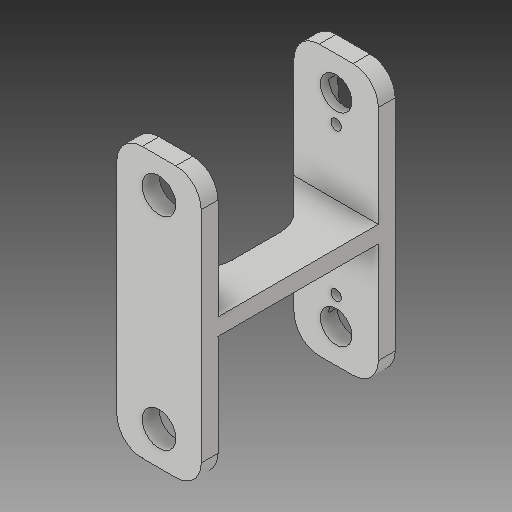
# Autodesk Inventor part: v5_femur
Saved by Autodesk Inventor 2019 (Build 230136000, 136)
## iProperties
Created: 2019-02-03
Part Number: v5_femur
Material: Generic
Document SubType Name: Modeling
Designer: Daniel
Density: 1 g/cm^3
Appearance: Default
Author: Daniel
Autodesk Inventor part; units mm, degrees
note: some values were not read from the file. Chosen so that the rebuilt part matches the saved one: direction of "Hole1"; direction of "Hole4"; direction of "Hole5"; direction of "Hole6"; direction of "Hole7".
ref_plane "YZ Plane" through (0, 0, 0) normal (1, 0, 0) x (0, 1, 0)
ref_plane "XZ Plane" through (0, 0, 0) normal (0, 1, 0) x (-1, 0, 0)
ref_plane "XY Plane" through (0, 0, 0) normal (0, 0, 1) x (1, 0, 0)
sketch "Sketch1" plane through (0, 0, 0) normal (0, 1, 0) x (-1, 0, 0)
  line L0 (14, 0) -> (-14, 0) projected
  line L1 (0, -32.2) -> (0, 32.2) projected
  line L2 (10, 23) -> (-10, 23)
  line L3 (-10, 23) -> (-10, -23)
  line L4 (-10, -23) -> (10, -23)
  line L5 (10, -23) -> (10, 23)
  point P0 (0, 0)
  dimension "d0" = 46
  dimension "d1" = 20
  constraints: 8 end point, 2 parallel, 1 horizontal, 1 perpendicular, 2 other
  measures "d0" distance between parallel lines of L4 L2
  measures "d1" distance between parallel lines of L3 L5
extrude "Extrusion1" add sketch "Sketch1" along normal blind 4
sketch "Sketch2" plane through (0, 4, 0) normal (0, 1, 0) x (1, 0, 0)
  line L0 (-10, -23) -> (10, -23) projected
  line L1 (10, -23) -> (10, 23) projected
  line L2 (10, 23) -> (-10, 23) projected
  line L3 (-10, 23) -> (-10, -23) projected
  line L4 (-10, -23) -> (10, -23)
  line L5 (10, -23) -> (10, -19)
  line L6 (10, -19) -> (-10, -19)
  line L7 (-10, -19) -> (-10, -23)
  line L8 (-10, 19) -> (10, 19)
  line L9 (10, 19) -> (10, 23)
  line L10 (10, 23) -> (-10, 23)
  line L11 (-10, 23) -> (-10, 19)
  line L12 (-10, -23) -> (10, -23) projected
  line L13 (-10, 23) -> (-10, -23) projected
  line L14 (10, -23) -> (10, 23) projected
  line L15 (10, 23) -> (-10, 23) projected
  point P0 (0, 0)
  dimension "d4" = 4
  dimension "d5" = 4
  constraints: 16 end point, 4 collinear, 4 parallel, 2 horizontal, 2 perpendicular, 2 point on line
  measures "d4" distance between parallel lines of L0 L6
  measures "d5" distance between parallel lines of L2 L8
extrude "Extrusion2" add sketch "Sketch2" along normal blind 30 contours L3 L6 L1 L0 | L3 L2 L1 L8
sketch "Sketch4" plane through (-10, 0, 23) normal (0, 0, 1) x (1, 0, 0)
  line L0 (0, 0) -> (20, 0) projected
  line L1 (20, 0) -> (20, 34) projected
  line L2 (0, 34) -> (20, 34) projected
  line L3 (0, 0) -> (0, 34) projected
  point P0 (10, 0)
  point P1 (10, 26)
  dimension "d8" = 10
  dimension "d9" = 8
  measures "d8" distance from line of L3 point (10, 26)
  measures "d9" distance from line of L2 point (10, 26)
hole "Hole1" at (0, 26, 23) direction (0, 0, -1) diameter 8 depth 42
sketch "Sketch10" plane through (10, 0, -23) normal (0, 0, -1) x (-1, 0, 0)
  line L0 (0, 34) -> (20, 34) projected
  line L1 (0, 0) -> (0, 34) projected
  line L2 (0, 0) -> (20, 0) projected
  line L3 (20, 0) -> (20, 34) projected
  circle A0 centre (10, 26) radius 4 projected
  circle A1 centre (10, 26) radius 3.75
  circle A2 centre (10, 12) radius 2.5
  line L4 (-6.7241, 9.5) -> (37.2046, 9.5) construction
  line L5 (6.25, 26) -> (7.5505, 11.5)
  line L6 (13.75, 26) -> (12.4495, 11.5)
  point P0 (10, 0)
  dimension "d47" = 16.5
  dimension "d48" = 7.5
  dimension "d49" = 5
  dimension "d50" = 10
  dimension "d51" = 2
  dimension "d52" = 2
  dimension "d53" = 8
  dimension "d54" = 8
  constraints: 6 end point, 4 point on circle, 2 centre point, 1 coincident, 1 horizontal, 1 tangent
  measures "d47" distance from line of L4 A1.centre
  measures "d48" diameter of A1
  measures "d49" diameter of A2
  measures "d50" distance from line of L1 A2.centre
  measures "d51" distance from line of L4 L6.end
  measures "d52" distance from line of L4 L5.end
  measures "d53" distance from line of L0 L6.start
  measures "d54" distance from line of L0 L5.start
extrude "Extrusion4" cut sketch "Sketch10" against normal blind 2 contours L5 A1 L6 A0 | A0 L6 A2 L5 | L5 A1 L6 | A2 L6 L5 picked at (10.4522, 22.2104)
sketch "Sketch11" plane through (10, 0, -21) normal (0, 0, -1) x (-1, 0, 0)
  line L0 (7.5505, 11.5) -> (6.25, 26) projected
  arc A0 (7.5505, 11.5) -> (12.4495, 11.5) centre (10, 12) ccw projected
  line L1 (13.75, 26) -> (12.4495, 11.5) projected
  arc A1 (13.75, 26) -> (6.25, 26) centre (10, 26) ccw projected
  point P0 (10, 0)
  constraints: 1 coincident
hole "Hole4" at (0, 26, -21) direction (0, 0, 1) diameter 7.5 depth 40
sketch "Sketch12" plane through (10, 0, -21) normal (0, 0, -1) x (-1, 0, 0)
  arc A0 (6.3099, 25.3327) -> (13.6901, 25.3327) centre (10, 26) ccw projected
  line L0 (7.5505, 11.5) -> (6.3099, 25.3327) projected
  arc A1 (7.5505, 11.5) -> (12.4495, 11.5) centre (10, 12) ccw projected
  line L1 (13.6901, 25.3327) -> (12.4495, 11.5) projected
  line L2 (0, 0) -> (0, 34) projected
  point P0 (10, 0)
  point P1 (10, 19.5)
  point P2 (0, 28)
  dimension "d64" = 6.5
  dimension "d65" = 10
  measures "d64" distance of A0.centre point (10, 19.5)
  measures "d65" distance from line of L2 point (10, 19.5)
hole "Hole5" at (0, 19.5, -21) direction (0, 0, 1) diameter 2.5 depth 40
sketch "Sketch13" plane through (0, 0, 0) normal (0, -1, 0) x (1, 0, 0)
  line L0 (-10, 23) -> (10, 23) projected
  line L1 (-10, -23) -> (-10, 23) projected
  line L2 (10, -23) -> (-10, -23) projected
  line L3 (10, 23) -> (10, -23) projected
  line L4 (10, 23) -> (10, -23) projected
  line L5 (-10, -19) -> (-10, 19) projected
  line L6 (10, 23) -> (-10, 23)
  line L7 (-10, 23) -> (-10, 19)
  line L8 (-10, 19) -> (10, 19)
  line L9 (10, 19) -> (10, 23)
  line L10 (10, -23) -> (-10, -23)
  line L11 (-10, -23) -> (-10, -19)
  line L12 (-10, -19) -> (10, -19)
  line L13 (10, -19) -> (10, -23)
  point P0 (0, 0)
  constraints: 16 end point, 4 parallel, 2 horizontal, 2 perpendicular
extrude "Extrusion5" add sketch "Sketch13" along normal blind 30 contours L0 L3 L8 L1 | L12 L3 L2 L1
sketch "Sketch14" plane through (10, 34, -23) normal (0, 0, -1) x (-1, 0, 0)
  arc A0 (7.5505, -22.5) -> (12.4495, -22.5) centre (10, -22) ccw projected
  line L0 (7.5505, -22.5) -> (6.25, -8) projected
  arc A1 (13.75, -8) -> (6.25, -8) centre (10, -8) ccw projected
  line L1 (13.75, -8) -> (12.4495, -22.5) projected
  line L2 (20, -64) -> (20, 0) projected
  line L3 (0, 0) -> (20, 0) projected
  line L4 (0, -64) -> (0, 0) projected
  line L5 (20, -64) -> (0, -64) projected
  line L6 (0, -34) -> (0, -64) projected
  line L7 (0, -40) -> (20, -40) construction
  circle A2 centre (10, -56) radius 3.75
  circle A3 centre (10, -42.5) radius 2.5
  line L8 (6.25, -56) -> (7.5505, -42)
  line L9 (13.75, -56) -> (12.4495, -42)
  point P0 (10, -34)
  dimension "d77" = 8
  dimension "d78" = 10
  dimension "d79" = 7.5
  dimension "d80" = 16
  dimension "d81" = 5
  dimension "d82" = 10
  dimension "d85" = 2
  dimension "d86" = 8
  dimension "d87" = 2
  dimension "d88" = 8
  constraints: 6 end point, 4 point on circle, 2 centre point, 2 point on line, 1 horizontal, 1 tangent
  measures "d77" distance from line of L5 A2.centre
  measures "d78" distance from line of L2 A2.centre
  measures "d79" diameter of A2
  measures "d80" distance from line of L7 A2.centre
  measures "d81" diameter of A3
  measures "d82" distance from line of L2 A3.centre
  measures "d85" distance from line of L7 L8.end
  measures "d86" distance from line of L5 L8.start
  measures "d87" distance from line of L7 L9.end
  measures "d88" distance from line of L5 L9.start
extrude "Extrusion6" cut sketch "Sketch14" against normal blind 2 contours L8 A2 L9 | L8 A3 L9 A2 | L8 A3 L9
sketch "Sketch15" plane through (10, 34, -21) normal (0, 0, -1) x (-1, 0, 0)
  arc A0 (6.25, -56) -> (13.75, -56) centre (10, -56) ccw projected
  line L0 (12.4495, -42) -> (13.75, -56) projected
  arc A1 (12.4495, -42) -> (7.5505, -42) centre (10, -42.5) ccw projected
  line L1 (6.25, -56) -> (7.5505, -42) projected
  point P0 (10, -34)
  constraints: 1 coincident
hole "Hole6" at (0, -22, -21) direction (0, 0, 1) diameter 7.5 depth 40
sketch "Sketch16" plane through (10, 34, -21) normal (0, 0, -1) x (-1, 0, 0)
  arc A0 (13.6858, -55.3093) -> (6.3142, -55.3093) centre (10, -56) ccw projected
  line L0 (12.4495, -42) -> (13.6858, -55.3093) projected
  arc A1 (12.4495, -42) -> (7.5505, -42) centre (10, -42.5) ccw projected
  line L1 (6.3142, -55.3093) -> (7.5505, -42) projected
  line L2 (12.4495, -42) -> (13.75, -56) projected
  arc A2 (6.25, -56) -> (13.75, -56) centre (10, -56) ccw projected
  line L3 (6.25, -56) -> (7.5505, -42) projected
  arc A3 (12.4495, -42) -> (7.5505, -42) centre (10, -42.5) ccw projected
  arc A4 (7.5505, -22.5) -> (12.4495, -22.5) centre (10, -22) ccw projected
  line L4 (7.5505, -22.5) -> (6.25, -8) projected
  arc A5 (13.75, -8) -> (6.25, -8) centre (10, -8) ccw projected
  line L5 (13.75, -8) -> (12.4495, -22.5) projected
  line L6 (20, -64) -> (20, 0) projected
  line L7 (0, 0) -> (20, 0) projected
  line L8 (0, -64) -> (0, 0) projected
  line L9 (20, -64) -> (0, -64) projected
  point P0 (10, -34)
  point P1 (10, -49.5)
  dimension "d98" = 10
  dimension "d99" = 6.5
  measures "d98" distance from line of L8 point (10, -49.5)
  measures "d99" distance of A0.centre point (10, -49.5)
hole "Hole7" at (0, -15.5, -21) direction (0, 0, 1) diameter 2.5 end up to surface
sketch "Sketch17" plane through (-10, 34, 23) normal (0, 0, 1) x (1, 0, 0)
  line L0 (20, -64) -> (0, -64) projected
  line L1 (20, -64) -> (20, 0) projected
  point P0 (10, -34)
  point P1 (10, -56)
  dimension "d107" = 8
  dimension "d108" = 10
  measures "d107" distance from line of L0 point (10, -56)
  measures "d108" distance from line of L1 point (10, -56)
hole "Hole8" at (0, -22, 23) direction (0, 0, -1) diameter 8 depth 4
fillet "Fillet4" radius 6 8 edges at (10, -30, -21) (-10, -30, -21) (10, -30, 21) (-10, -30, 21) (10, 34, 21) (10, 34, -21) (-10, 34, -21) (-10, 34, 21)
sketch "Sketch19" plane through (0, 0, 0) normal (0, -1, 0) x (1, 0, 0)
  line L0 (10, 19) -> (-10, 19) projected
  line L1 (-10, -19) -> (-10, 19) projected
  line L2 (-10, -19) -> (10, -19) projected
  line L3 (10, 19) -> (10, -19) projected
  line L4 (-10, -19) -> (-10, 19) projected
  line L5 (10, 19) -> (-10, 19) projected
  line L6 (-10, -19) -> (0, -19)
  line L7 (0, -19) -> (0, 19)
  line L8 (0, 19) -> (-10, 19)
  line L9 (-10, 19) -> (-10, -19)
  point P0 (0, 0)
  constraints: 8 end point, 2 parallel, 1 horizontal, 1 midpoint, 1 perpendicular
extrude "Extrusion8" cut sketch "Sketch19" against normal up to next contours L7 L2 L1 L0
chamfer "Chamfer1" distance 10 angle 45 2 edges at (0, 2, -19) (0, 2, 19)
fillet "Fillet6" radius 8 2 edges at (0, 2, 9) (0, 2, -9)
body "Solid1"
